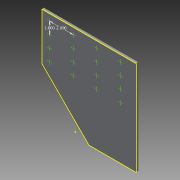
# Autodesk Inventor part: 2040-2040_mounting_plate
Saved by Autodesk Inventor 2014 (Build 180170000, 170)
## iProperties
Created: 2014-09-28
Part Number: 2040-2040_mounting_plate
Material: Generic
Document SubType Name: Modeling
Designer: Matthew
Density: 1 g/cm^3
Appearance: Default
Author: Matthew
Autodesk Inventor part; units mm, degrees
ref_plane "YZ Plane" through (0, 0, 0) normal (1, 0, 0) x (0, 1, 0)
ref_plane "XZ Plane" through (0, 0, 0) normal (0, 1, 0) x (-1, 0, 0)
ref_plane "XY Plane" through (0, 0, 0) normal (0, 0, 1) x (1, 0, 0)
sketch "Sketch1" plane through (0, 0, 0) normal (0, 0, 1) x (1, 0, 0)
  line L0 (-72.7046, 193.4128) -> (-72.7046, 91.8128)
  line L1 (-72.7046, 193.4128) -> (130.4954, 193.4128)
  line L2 (130.4954, 193.4128) -> (130.4954, -9.7872)
  line L3 (130.4954, -9.7872) -> (28.8954, -9.7872)
  line L4 (28.8954, -9.7872) -> (-72.7046, 91.8128)
  point P0 (0, 0)
  dimension "d0" = 101.6
  dimension "d1" = 101.6
  dimension "d2" = 203.2
  dimension "d3" = 203.2
  constraints: 10 end point, 2 perpendicular, 1 parallel, 1 vertical
  measures "d0" distance of L0.start L0.end
  measures "d1" distance of L2.end L3.end
  measures "d2" distance of L0.start L1.end
  measures "d3" distance of L1.end L2.end
extrude "Extrusion1" add sketch "Sketch1" along normal blind 4.7625
sketch "Sketch2" plane through (0, 0, 4.7625) normal (0, 0, 1) x (1, 0, 0)
  line L0 (-72.7046, 193.4128) -> (-72.7046, 91.8128) projected
  line L1 (28.8954, -9.7872) -> (130.4954, -9.7872) projected
  line L2 (130.4954, -9.7872) -> (130.4954, 193.4128) projected
  line L3 (130.4954, 193.4128) -> (-72.7046, 193.4128) projected
  point P0 (0, 0)
  point P1 (-60.0046, 180.7128)
  point P2 (-34.6046, 180.7128)
  point P3 (-60.0046, 155.3128)
  point P4 (-34.6046, 155.3128)
  point P5 (-60.0046, 129.9128)
  point P6 (-34.6046, 129.9128)
  point P7 (-60.0046, 104.5128)
  point P8 (-34.6046, 104.5128)
  point P9 (117.7954, 79.1128)
  point P10 (117.7954, 53.7128)
  point P11 (92.3954, 79.1128)
  point P12 (92.3954, 53.7128)
  point P13 (-9.2046, 180.7128)
  point P14 (-9.2046, 155.3128)
  point P15 (-9.2046, 129.9128)
  point P16 (-9.2046, 104.5128)
  point P17 (16.1954, 180.7128)
  point P18 (16.1954, 155.3128)
  point P19 (16.1954, 129.9128)
  point P20 (16.1954, 104.5128)
  point P21 (41.5954, 180.7128)
  point P22 (41.5954, 155.3128)
  point P23 (41.5954, 129.9128)
  point P24 (41.5954, 104.5128)
  point P25 (66.9954, 180.7128)
  point P26 (66.9954, 155.3128)
  point P27 (66.9954, 129.9128)
  point P28 (66.9954, 104.5128)
  point P29 (92.3954, 180.7128)
  point P30 (92.3954, 155.3128)
  point P31 (92.3954, 129.9128)
  point P32 (92.3954, 104.5128)
  point P33 (117.7954, 180.7128)
  point P34 (117.7954, 155.3128)
  point P35 (117.7954, 129.9128)
  point P36 (117.7954, 104.5128)
  point P37 (117.7954, 28.3128)
  point P38 (92.3954, 28.3128)
  point P39 (117.7954, 2.9128)
  point P40 (92.3954, 2.9128)
  point P41 (66.9954, 79.1128)
  point P42 (66.9954, 53.7128)
  point P43 (66.9954, 28.3128)
  point P44 (66.9954, 2.9128)
  point P45 (41.5954, 79.1128)
  point P46 (41.5954, 53.7128)
  point P47 (41.5954, 28.3128)
  point P48 (41.5954, 2.9128)
  dimension "d8" = 25.4
  dimension "d11" = 25.4
  dimension "d17" = 25.4
  dimension "d20" = 25.4
  dimension "d26" = 12.7
  dimension "d27" = 12.7
  dimension "d28" = 25.4
  constraints: 2 horizontal, 2 vertical, 1 vertical alignment, 46 other
  measures "d8" distance of point (-60.005, 180.713) point (-34.605, 180.713)
  measures "d11" distance of point (-60.005, 180.713) point (-60.005, 155.313)
  measures "d17" distance of point (117.795, 79.113) point (117.795, 53.713)
  measures "d20" distance of point (117.795, 79.113) point (92.395, 79.113)
  measures "d26" distance from line of L3 point (-34.605, 180.713)
  measures "d27" distance from line of L0 point (-60.005, 180.713)
  measures "d28" distance of point (117.795, 104.513) point (117.795, 79.113)
hole "Hole1" at (-60.0046, 180.7128, 4.7625) at (-34.6046, 180.7128, 4.7625) at (-60.0046, 155.3128, 4.7625) at (-34.6046, 155.3128, 4.7625) at (-60.0046, 129.9128, 4.7625) at (-34.6046, 129.9128, 4.7625) at (-60.0046, 104.5128, 4.7625) at (-34.6046, 104.5128, 4.7625) at (117.7954, 79.1128, 4.7625) at (117.7954, 53.7128, 4.7625) at (92.3954, 79.1128, 4.7625) at (92.3954, 53.7128, 4.7625) at (-9.2046, 180.7128, 4.7625) at (-9.2046, 155.3128, 4.7625) at (-9.2046, 129.9128, 4.7625) at (-9.2046, 104.5128, 4.7625) at (16.1954, 180.7128, 4.7625) at (16.1954, 155.3128, 4.7625) at (16.1954, 129.9128, 4.7625) at (16.1954, 104.5128, 4.7625) at (41.5954, 180.7128, 4.7625) at (41.5954, 155.3128, 4.7625) at (41.5954, 129.9128, 4.7625) at (41.5954, 104.5128, 4.7625) at (66.9954, 180.7128, 4.7625) at (66.9954, 155.3128, 4.7625) at (66.9954, 129.9128, 4.7625) at (66.9954, 104.5128, 4.7625) at (92.3954, 180.7128, 4.7625) at (92.3954, 155.3128, 4.7625) at (92.3954, 129.9128, 4.7625) at (92.3954, 104.5128, 4.7625) at (117.7954, 180.7128, 4.7625) at (117.7954, 155.3128, 4.7625) at (117.7954, 129.9128, 4.7625) at (117.7954, 104.5128, 4.7625) at (117.7954, 28.3128, 4.7625) at (92.3954, 28.3128, 4.7625) at (117.7954, 2.9128, 4.7625) at (92.3954, 2.9128, 4.7625) at (66.9954, 79.1128, 4.7625) at (66.9954, 53.7128, 4.7625) at (66.9954, 28.3128, 4.7625) at (66.9954, 2.9128, 4.7625) at (41.5954, 79.1128, 4.7625) at (41.5954, 53.7128, 4.7625) at (41.5954, 28.3128, 4.7625) at (41.5954, 2.9128, 4.7625) direction (0, 0, -1) diameter 6.35 end through all
equation "\"d1\" = d0"
equation "\"d3\" = d2"
body "Solid1"
